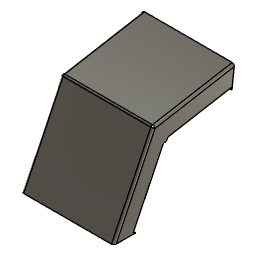
指甲刀主体 v16 (Autodesk Fusion 360 archive; units mm, degrees)
design "撑脚"
Autodesk Fusion 360 part; units mm, degrees
sketch "草图1" plane through (0, 0, 0) normal (1, 0, 0) x (0, 1, 0)
  line L0 (-83.2313, 7.1) -> (-98.0035, 4.4953)
  line L1 (-83.2313, 7.1) -> (-68.15, 7.1) construction
  line L2 (-98.0035, 4.4953) -> (-104.9367, -9.9245)
  line L3 (-104.9367, -9.9245) -> (-109.9947, -9.9245)
  line L4 (-83.2313, 7.1) -> (-82.6393, 12.0648)
  line L5 (-83.2313, 7.1) -> (-78.15, 7.1) construction
  line L6 (-82.6393, 12.0648) -> (-100.9782, 8.8312)
  line L7 (-109.9947, -9.9245) -> (-100.9765, 8.8315)
  dimension "d1" = 170
  dimension "d2" = 15
  dimension "d3" = 16
  dimension "d4" = 83.2
  dimension "d5" = 5
  constraint horizontal L1
  constraint horizontal L3
  constraint horizontal L5
  constraint parallel L0 L6
  constraint parallel L2 L7
  constraint coincident L6 L7.end
  measures "d1" angle of L0 L1
  measures "d2" distance of L0.start L0.end
  measures "d3" distance of L0.end L2.end
  measures "d4" angle of L4 L5
  measures "d5" distance of L0.start L4.end
extrude "拉伸1" add sketch "草图1" against normal blind 10
extrude "拉伸2" add 1 faces at (-10, -93.8737, 8.4638) along direction (-1, 0, 0) blind 15
move_body "移动1" bodies 1 to x (1, 0, 0) y (0, 1, 0) z (0, 0, 1) at (-12.5, 0, 0)
extrude "拉伸3" cut 1 faces at (-37.5, -93.8737, 8.4638) along direction (1, 0, 0) blind 2
extrude "拉伸4" cut 1 faces at (-12.5, -93.8737, 8.4638) along direction (-1, 0, 0) blind 2
move_body "移动2" bodies 1 to x (1, 0, 0) y (0, 1, 0) z (0, 0, 1) at (0, -16, 0)
extrude "拉伸5" cut 1 faces at (-14.5, -109.8737, 8.4638) along direction (-1, 0, 0) blind 0.1
extrude "拉伸6" cut 1 faces at (-35.5, -109.8737, 8.4638) along direction (1, 0, 0) blind 0.1
extrude "拉伸7" cut 1 faces at (-21.5333, -104.7523, 10.9869) along direction (0, 0.173648, -0.984808) blind 0.1
extrude "拉伸8" cut 1 faces at (-21.5333, -119.9837, 2.5793) along direction (0, 0.901237, -0.433326) blind 0.1
extrude "拉伸9" cut 1 faces at (-21.5333, -104.1554, 6.2318) along direction (0, -0.173648, 0.984808) blind 0.1
extrude "拉伸10" cut 1 faces at (-28.4667, -118.6256, -5.1179) along direction (0, -0.901237, 0.433326) blind 0.1
fillet "圆角1" radius 0.5 1 edges at (-14.6, -107.7802, 10.3515)
fillet "圆角2" radius 0.5 1 edges at (-35.4, -107.7802, 10.3515)
fillet "圆角3" radius 1 1 edges at (-25, -114.0035, 4.4953)
fillet "圆角4" radius 0.5 1 edges at (-35.4, -106.6348, 5.8961)
fillet "圆角5" radius 0.5 1 edges at (-35.4, -117.5602, -2.6713)
fillet "圆角6" radius 0.5 1 edges at (-14.6, -106.6348, 5.8961)
fillet "圆角7" radius 0.5 1 edges at (-14.6, -117.5602, -2.6713)
fillet "圆角8" radius 0.5 5 edges at (-35.4, -121.5295, -0.8687) (-35.2536, -116.9868, 8.5794) (-25, -116.9086, 8.7419) (-14.7464, -116.9868, 8.5794) (-14.6, -121.5295, -0.8687)

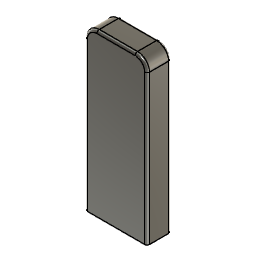
design "推杆橡胶套"
Autodesk Fusion 360 part; units mm, degrees
sketch "草图1" plane through (0, 0, 0) normal (0, 0, 1) x (1, 0, 0)
  line L0 (-122.5473, -24.9077) -> (-143.5473, -24.9077)
  line L1 (-143.5473, -24.9077) -> (-143.5473, -19.9077)
  line L2 (-143.5473, -19.9077) -> (-122.5473, -19.9077)
  line L3 (-122.5473, -19.9077) -> (-122.5473, -24.9077)
  line L4 (-146.0473, -17.4077) -> (-120.0473, -17.4077)
  line L5 (-120.0473, -17.4077) -> (-120.0473, -27.4077)
  line L6 (-120.0473, -27.4077) -> (-146.0473, -27.4077)
  line L7 (-146.0473, -27.4077) -> (-146.0473, -17.4077)
  line L8 (-146.0473, -17.4077) -> (-120.0473, -27.4077) construction
  line L9 (-120.0473, -17.4077) -> (-146.0473, -27.4077) construction
  point P0 (-133.0473, -22.4077)
  dimension "d1" = 21
  dimension "d2" = 5
  dimension "d3" = 26
  dimension "d4" = 10
  constraint horizontal L0
  constraint vertical L1
  constraint horizontal L2
  constraint vertical L3
  constraint horizontal L4
  constraint perpendicular L4 L5
  constraint parallel L4 L6
  constraint parallel L5 L7
  constraint coincident L8 P0
  constraint coincident L9 P0
  measures "d1" distance of L0.start L0.end
  measures "d2" distance of L0.start L2.end
  measures "d3" distance of L5.end L6.end
  measures "d4" distance of L4.end L5.end
extrude "拉伸1" add sketch "草图1" along normal blind 65
sketch "草图2" plane through (0, 0, 65) normal (0, 0, 1) x (-1, 0, 0)
  line L0 (143.5473, 19.9077) -> (122.5473, 19.9077)
  line L1 (122.5473, 19.9077) -> (122.5473, 24.9077)
  line L2 (122.5473, 24.9077) -> (143.5473, 24.9077)
  line L3 (143.5473, 24.9077) -> (143.5473, 19.9077)
  line L4 (146.0473, 27.4077) -> (120.0473, 27.4077)
  line L5 (120.0473, 27.4077) -> (120.0473, 17.4077)
  line L6 (120.0473, 17.4077) -> (146.0473, 17.4077)
  line L7 (146.0473, 17.4077) -> (146.0473, 27.4077)
  line L8 (120.0473, 27.4077) -> (146.0473, 27.4077)
  line L9 (146.0473, 27.4077) -> (146.0473, 17.4077)
  line L10 (146.0473, 17.4077) -> (120.0473, 17.4077)
  line L11 (120.0473, 17.4077) -> (120.0473, 27.4077)
  constraint horizontal L8
  constraint vertical L9
  constraint horizontal L10
  constraint vertical L11
  constraint coincident L6.end L7.start
  constraint coincident L4.end L5.start
extrude "拉伸2" add sketch "草图2" along normal blind 2.5 contours L0 L1 L2 L3 | L4 L5 L6 L7 L8 L9 L10 L11
fillet "圆角1" radius 5 1 edges at (-122.5473, -22.4077, 65)
fillet "圆角2" radius 5 1 edges at (-143.5473, -22.4077, 65)
fillet "圆角3" radius 5 1 edges at (-120.0473, -22.4077, 67.5)
fillet "圆角4" radius 5 1 edges at (-146.0473, -22.4077, 67.5)
fillet "圆角5" radius 1 5 edges at (-120.0473, -17.4077, 31.25) (-121.5118, -17.4077, 66.0355) (-133.0473, -17.4077, 67.5) (-144.5829, -17.4077, 66.0355) (-146.0473, -17.4077, 31.25)
fillet "圆角6" radius 1 5 edges at (-146.0473, -27.4077, 31.25) (-144.5829, -27.4077, 66.0355) (-133.0473, -27.4077, 67.5) (-121.5118, -27.4077, 66.0355) (-120.0473, -27.4077, 31.25)
